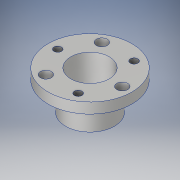
# Autodesk Inventor part: Torch Holder Upper
Saved by Autodesk Inventor 2018.2 (Build 222227000, 227)
## iProperties
Created: 2018-03-02
Part Number: Torch Holder Upper
Material: Aluminum 6061
Document SubType Name: Modeling
Designer: torba
Density: 2.7 g/cm^3
Appearance: Aluminum - Flat
Author: torba
Autodesk Inventor part; units mm, degrees
ref_plane "YZ Plane" through (0, 0, 0) normal (1, 0, 0) x (0, 1, 0)
ref_plane "XZ Plane" through (0, 0, 0) normal (0, 1, 0) x (-1, 0, 0)
ref_plane "XY Plane" through (0, 0, 0) normal (0, 0, 1) x (1, 0, 0)
sketch "Sketch1" plane through (0, 0, 0) normal (0, 1, 0) x (-1, 0, 0)
  arc A0 (90.342, -38.2341) -> (90.342, 35.0591) centre (100.765, -1.5875) ccw
  circle A1 centre (100.765, -1.5875) radius 38.1
  line L0 (100.765, -1.5875) -> (138.865, -1.5875) construction
  line L1 (100.765, -1.5875) -> (81.715, -34.5831) construction
  line L2 (100.765, -1.5875) -> (138.865, -1.5875) construction
  line L3 (100.765, -1.5875) -> (81.715, 31.4081) construction
  line L4 (100.765, -1.5875) -> (138.865, -1.5875) construction
  circle A2 centre (100.765, -1.5875) radius 29.3687 construction
  circle A3 centre (100.765, -1.5875) radius 17.4625
  point P0 (115.4494, 23.8466)
  point P1 (115.4494, -27.0216)
  point P2 (71.3963, -1.5875)
  dimension "d0" = 120
  dimension "d1" = 120
  dimension "d12" = 34.925
  constraints: 10 end point, 6 point on circle, 3 centre point, 2 coincident, 2 equal length, 2 horizontal, 1 concentric, 3 other
  measures "d0" angle of L1 L2
  measures "d1" angle of L4 L3
  measures "d12" diameter of A3
extrude "Extrusion1" add sketch "Sketch1" along normal blind 9.525
hole "Hole1" at (-115.4494, 0, 23.8466) at (-115.4494, 0, -27.0216) at (-71.3963, 0, -1.5875) direction (0, 1, 0) diameter 10 depth 9.525 tip angle 118
sketch "Sketch2" plane through (-100.765, 0, -1.5875) normal (0, -1, 0) x (1, 0, 0)
  circle A0 centre (0, 0) radius 17.4625 projected
  line L0 (0, 17.4625) -> (0, 22.225)
  circle A1 centre (0, 0) radius 22.225
  point P0 (100.765, 1.5875)
  dimension "d22" = 4.7625
  constraints: 2 end point, 2 vertical alignment, 1 coincident, 1 vertical, 3 other
  measures "d22" distance of L0.start L0.end
extrude "Extrusion2" add sketch "Sketch2" along normal blind 25.4
sketch "Sketch3" plane through (-100.765, 0, -1.5875) normal (0, -1, 0) x (1, 0, 0)
  circle A0 centre (0, 0) radius 38.1 projected
  circle A1 centre (29.3687, 0) radius 5 projected
  circle A2 centre (0, 0) radius 29.3687
  line L0 (0, 0) -> (14.6844, -25.4341)
  line L1 (0, 0) -> (29.3687, 0) construction
  line L2 (0, 0) -> (-29.3687, 0)
  line L3 (0, 0) -> (14.6844, 25.4341)
  line L4 (0, 0) -> (29.3687, 0) construction
  point P0 (100.765, 1.5875)
  dimension "d26" = 60
  dimension "d27" = 60
  constraints: 10 end point, 4 coincident, 4 point on circle, 3 horizontal, 2 equal length, 1 centre point
  measures "d26" angle of L0 L1
  measures "d27" angle of L4 L3
hole "Hole2" at (-86.0806, 0, 23.8466) at (-86.0806, 0, -27.0216) at (-130.1337, 0, -1.5875) direction (0, 1, 0) diameter 6.9088 depth 21.1074 tip angle 118
body "Solid1"
